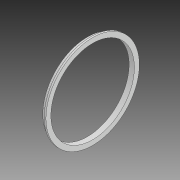
# Autodesk Inventor part: SwivelMountClamp
Saved by Autodesk Inventor 2020 (Build 240168000, 168)
## iProperties
Created: 2020-09-19
Part Number: SwivelMountClamp
Material: Generic
Document SubType Name: Modeling
Designer: DDeGo
Density: 1 g/cm^3
Appearance: Default
Author: DDeGo
Autodesk Inventor part; units mm, degrees
ref_plane "YZ Plane" through (0, 0, 0) normal (1, 0, 0) x (0, 1, 0)
ref_plane "XZ Plane" through (0, 0, 0) normal (0, 1, 0) x (-1, 0, 0)
ref_plane "XY Plane" through (0, 0, 0) normal (0, 0, 1) x (1, 0, 0)
sketch "Sketch1" plane through (0, 0, 0) normal (0, 0, 1) x (1, 0, 0)
  line L0 (0, 0) -> (0, -59.4) construction
  line L1 (0, -59.4) -> (7.5, -59.4)
  line L2 (7.5, -59.4) -> (7.5, -66.4)
  line L3 (7.5, -66.4) -> (5, -66.4)
  line L4 (5, -66.4) -> (5, -63.4)
  line L5 (5, -63.4) -> (0, -63.4)
  line L6 (0, -63.4) -> (0, -59.4)
  line L7 (0, 0) -> (7.5, 0) construction
  line L8 (7.5, 0) -> (7.5, -59.4) construction
  line L9 (7.5, -59.4) -> (7.5, -66.4)
  dimension "d0" = 63.4
  dimension "d1" = 4
  dimension "d2" = 2.5
  dimension "d3" = 3
  dimension "d4" = 5
  constraints: 20 end point, 7 perpendicular, 1 coincident, 1 collinear, 1 horizontal, 1 point on line, 1 vertical
  measures "d0" distance from line of L7.start L5
  measures "d1" distance between parallel lines of L1 L5
  measures "d2" distance between parallel lines of L2 L4
  measures "d3" distance of L3.end L4.end
  measures "d4" distance of L4.end L5.end
revolve "Revolution1" add sketch "Sketch1" angle 360 about axis through (0, 0, 0) along (1, 0, 0)
body "Solid1"
